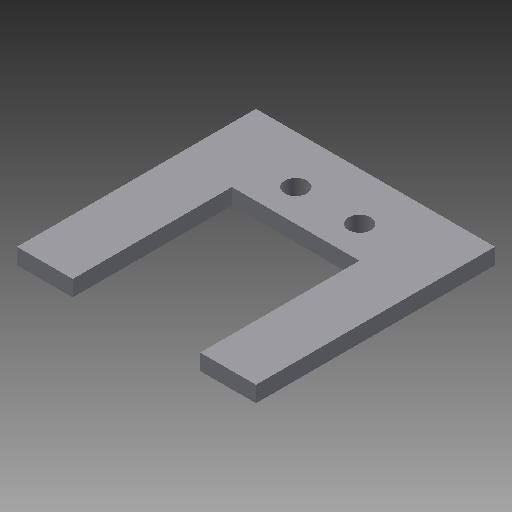
# Autodesk Inventor part: Shutter
Saved by Autodesk Inventor 2018 (Build 220112000, 112)
## iProperties
Created: 2015-02-10
Part Number: Shutter
Material: Generic
Document SubType Name: Modeling
Designer: Pascal
Density: 1 g/cm^3
Appearance: Default
Author: Pascal
Autodesk Inventor part; units mm, degrees
ref_plane "YZ Plane" through (0, 0, 0) normal (1, 0, 0) x (0, 1, 0)
ref_plane "XZ Plane" through (0, 0, 0) normal (0, 1, 0) x (-1, 0, 0)
ref_plane "XY Plane" through (0, 0, 0) normal (0, 0, 1) x (1, 0, 0)
sketch "Sketch1" plane through (0, 0, 0) normal (0, 1, 0) x (-1, 0, 0)
  line L0 (9.211, 8.9923) -> (-9.839, 8.9923)
  line L1 (-9.839, 8.9923) -> (-9.839, -10.0577)
  line L2 (-9.839, -10.0577) -> (9.211, -10.0577)
  line L3 (9.211, -10.0577) -> (9.211, 8.9923)
  point P0 (0, 0)
  dimension "d0" = 19.05
  dimension "d1" = 19.05
  constraints: 8 end point, 2 parallel, 1 horizontal, 1 perpendicular
  measures "d0" distance of L2.end L0.start
  measures "d1" distance of L1.end L2.end
extrude "Extrusion1" add sketch "Sketch1" along normal blind 1.27
sketch "Sketch2" plane through (0, 1.27, 0) normal (0, 1, 0) x (1, 0, 0)
  line L0 (-4.766, -9.0074) -> (5.394, -9.0074)
  line L1 (5.394, -9.0074) -> (5.394, 3.6926)
  line L2 (5.394, 3.6926) -> (-4.766, 3.6926)
  line L3 (-4.766, 3.6926) -> (-4.766, -9.0074)
  line L4 (-9.211, 10.0577) -> (-9.211, -8.9923) projected
  point P0 (0, 0)
  dimension "d4" = 4.445
  dimension "d5" = 10.16
  dimension "d6" = 12.7
  constraints: 8 end point, 2 parallel, 1 horizontal, 1 perpendicular
  measures "d4" distance between parallel lines of L3 L4
  measures "d5" distance between parallel lines of L1 L3
  measures "d6" distance of L2.end L0.start
extrude "Extrusion2" cut sketch "Sketch2" against normal up to next
hole "Hole1" at (-2.226, 1.27, -6.2477) direction (0, -1, 0) diameter 1.778 depth 1.27 clearance for "Flat Head Machine Screw (82)" size "#0" standard "Ansi Unified Screw Threads"
hole "Hole2" at (2.854, 1.27, -6.2477) direction (0, -1, 0) diameter 1.778 depth 1.27 clearance for "Flat Head Machine Screw (82)" size "#0" standard "Ansi Unified Screw Threads"
body "Solid1"
